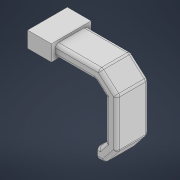
# Autodesk Inventor part: Verbindung_Motor_Servo_v2
Saved by Autodesk Inventor 2021 (Build 250183000, 183)
## iProperties
Created: 2021-01-05
Part Number: Verbindung_Motor_Servo_v2
Material: Generisch
Document SubType Name: Modeling
Designer: laure
Density: 1 g/cm^3
Appearance: Vorgabe
Author: laure
Autodesk Inventor part; units mm, degrees
ref_plane "YZ Plane" through (0, 0, 0) normal (1, 0, 0) x (0, 1, 0)
ref_plane "XZ Plane" through (0, 0, 0) normal (0, 1, 0) x (-1, 0, 0)
ref_plane "XY Plane" through (0, 0, 0) normal (0, 0, 1) x (1, 0, 0)
sketch "Skizze1" plane through (0, 0, 0) normal (0, 1, 0) x (-1, 0, 0)
  line L0 (15, 25) -> (-15, 25)
  line L1 (-15, 25) -> (-15, -25)
  line L2 (-15, -25) -> (15, -25)
  line L3 (15, -25) -> (15, 25)
  line L4 (0, -35) -> (0, 35) projected
  line L5 (-21, 0) -> (21, 0) projected
  point P0 (0, 0)
  dimension "d0" = 50
  dimension "d1" = 30
  constraints: 8 end point, 2 parallel, 1 horizontal, 1 perpendicular, 2 other
  measures "d0" distance of L2.end L0.start
  measures "d1" distance of L1.end L2.end
extrude "Extrusion1" add sketch "Skizze1" along normal mid plane 20
sketch "Skizze2" plane through (15, -10, -25) normal (1, 0, 0) x (0, 0, -1)
  line L0 (-60, 10) -> (10, 10) projected
  line L1 (-25, -4) -> (-25, 24) projected
  line L2 (-45, 17) -> (-5, 17)
  line L3 (-5, 17) -> (-5, 3)
  line L4 (-5, 3) -> (-45, 3)
  line L5 (-45, 3) -> (-45, 17)
  point P0 (-25, 10)
  dimension "d4" = 40
  dimension "d5" = 14
  constraints: 8 end point, 2 parallel, 1 horizontal, 1 perpendicular, 2 other
  measures "d4" distance of L2.start L2.end
  measures "d5" distance of L2.end L3.end
sketch "Skizze3" plane through (0, 0, 0) normal (0, 0, 1) x (1, 0, 0)
  line L0 (-21, 0) -> (21, 0) projected
  line L1 (0, 14) -> (0, -14) projected
  line L2 (15, -10) -> (15, 10) projected
  line L3 (15, 0) -> (68, 0)
  line L4 (85, -15) -> (85, -70)
  line L5 (85, -70) -> (73, -85)
  line L6 (73, -85) -> (68, -85)
  line L7 (15, -14) -> (15, 14) projected
  line L8 (85, -15) -> (68, 0)
  point P0 (0, 0)
  dimension "d16" = 68
  dimension "d17" = 53
  dimension "d18" = 85
  dimension "d19" = 85
  dimension "d20" = 55
  dimension "d21" = 5
  dimension "d22" = 53
  dimension "d23" = 15
  constraints: 10 end point, 1 midpoint, 1 perpendicular, 1 point on line, 1 vertical
  measures "d16" distance from line of L6.end L1
  measures "d17" distance from line of L6.end L7
  measures "d18" distance between parallel lines of L1 L4
  measures "d19" distance between parallel lines of L6 L3
  measures "d20" distance of L4.start L4.end
  measures "d21" distance of L5.end L6.end
  measures "d22" distance of L3.start L3.end
  measures "d23" vertical distance of L4.start L3.end
sweep "Sweeping1" add profiles "Skizze2" path "Skizze3" path curves L3 L8 L4 L5 L6
fillet "Rundung1" radius 4 1 edges at (42.8234, 7, -20)
fillet "Rundung2" radius 4 3 edges at (71.9745, 5.8284, -18.8284) (83.59, -4.4206, -20) (70.6467, 7, 2)
fillet "Rundung3" radius 4 3 edges at (70.549, 6.7415, 20) (81.8904, -2.9209, 20) (42.0672, 7, 20)
fillet "Rundung4" radius 4 12 edges at (40.1766, -7, -20) (65.3533, -7, 0) (40.1766, -7, 20) (71.6766, -12.5794, -20) (78, -42.8517, -20) (92, -13.4036, -18.8284) (92, -11.8411, 0) (92, -13.4036, 18.8284) (92, -44.8155, 20) (92, -44.8155, -20) (71.6766, -12.5794, 20) (78, -42.8517, 20)
fillet "Rundung5" radius 4 5 edges at (90.8284, -73.9199, -18.8284) (92, -72.4555, 0) (90.8284, -73.9199, 18.8284) (82.1822, -84.7277, 20) (82.1822, -84.7277, -20)
fillet "Rundung6" radius 4 5 edges at (74.864, -92, 18.8284) (69.6209, -92, 20) (74.864, -92, -18.8284) (69.6209, -92, -20) (76.3644, -92, 0)
fillet "Rundung7" radius 4 2 edges at (75.8178, -70.2723, -20) (75.8178, -70.2723, 20)
fillet "Rundung8" radius 4 2 edges at (71.3791, -78, -20) (71.3791, -78, 20)
fillet "Rundung9" radius 4 6 edges at (79.1716, -67.9555, -18.8284) (79.1716, -67.9555, 18.8284) (78, -67.5445, 0) (79.1716, -17.6302, -18.8284) (79.1716, -17.6302, 18.8284) (78, -18.1589, 0)
